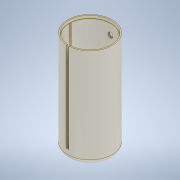
# Autodesk Inventor part: Exterior
Saved by Autodesk Inventor 2020 (Build 240168000, 168)
## iProperties
Created: 2020-10-28
Part Number: Exterior
Material: ABS Plastic
Document SubType Name: Modeling
Designer: aaron
Density: 1.06 g/cm^3
Appearance: Titanium - Polished
Author: aaron
Autodesk Inventor part; units mm, degrees
ref_plane "YZ Plane" through (0, 0, 0) normal (1, 0, 0) x (0, 1, 0)
ref_plane "XZ Plane" through (0, 0, 0) normal (0, 1, 0) x (-1, 0, 0)
ref_plane "XY Plane" through (0, 0, 0) normal (0, 0, 1) x (1, 0, 0)
sketch "Sketch1" plane through (0, 0, 0) normal (0, 0, 1) x (1, 0, 0)
  line L0 (0, 0) -> (35, 0)
  line L1 (45, 10) -> (45, 200)
  line L2 (0, 200) -> (0, 0)
  arc A0 (35, 0) -> (45, 10) centre (35, 10) ccw
  line L3 (41.5, 200) -> (41.5, 10)
  arc A1 (35, 3.5) -> (41.5, 10) centre (35, 10) ccw
  line L4 (35, 3.5) -> (0, 3.5)
  line L5 (41.5, 200) -> (45, 200)
  line L6 (0, 3.5) -> (0, 0)
  point P0 (45, 0)
  dimension "d0" = 90
  dimension "d1" = 200
  dimension "d2" = 10
  dimension "d5" = 3.5
  dimension "d6" = 3.5
  constraints: 14 end point, 4 point on circle, 3 point on line, 2 centre point, 2 horizontal, 2 perpendicular, 2 tangent, 2 vertical, 1 other
  measures "d0" diameter of L1 L2
  measures "d1" distance of point (45, 0) L1.end
  measures "d2" radius of A0
  measures "d5" distance between parallel lines of L0 L4
  measures "d6" distance between parallel lines of L1 L3
revolve "Revolution1" add sketch "Sketch1" angle 360 about axis through (0, 200, 0) along (0, -1, 0)
sketch "Sketch2" plane through (0, 200, 0) normal (0, 1, 0) x (1, 0, 0)
  circle A0 centre (0, 0) radius 45 construction
  line L0 (0, 45) -> (0, -45) construction
  line L1 (-45, 0) -> (45, 0) construction
  circle A1 centre (0, 0) radius 45 construction
  circle A2 centre (0, 0) radius 41.5 construction
  circle A3 centre (0, 0) radius 41.5 construction
  circle A4 centre (0, 0) radius 45 construction
  line L2 (0, -41.5) -> (0, -45) construction
  line L3 (-2.5, -45.45) -> (2.5, -45.45)
  line L4 (2.5, -45.45) -> (2.5, -41.05)
  line L5 (2.5, -41.05) -> (-2.5, -41.05)
  line L6 (-2.5, -41.05) -> (-2.5, -45.45)
  line L7 (-2.5, -45.45) -> (2.5, -41.05) construction
  line L8 (2.5, -45.45) -> (-2.5, -41.05) construction
  point P0 (0, -43.25)
  dimension "d8" = 5
  dimension "d9" = 4.4
  constraints: 18 end point, 4 point on circle, 3 midpoint, 2 parallel, 2 perpendicular, 1 collinear, 1 point on line, 1 vertical, 1 vertical alignment, 1 other
  measures "d8" distance of L3.start L3.end
  measures "d9" distance of L3.end L4.end
extrude "Extrusion1" cut sketch "Sketch2" against normal blind 180
fillet "Fillet1" radius 1 2 edges at (-2.5, 200, 43.1776) (2.5, 200, 43.1776)
sketch "Sketch3" plane through (0, 200, 0) normal (0, 1, 0) x (1, 0, 0)
  arc A0 (3.5, -41.3521) -> (-3.5, -41.3521) centre (0, 0) ccw projected
  circle A1 centre (0, 0) radius 42.5
  circle A2 centre (0, 0) radius 41.5
  point P0 (3.5, -41.3521)
  point P1 (-3.5, -41.3521)
  dimension "d13" = 85
  constraints: 2 centre point, 2 coincident, 1 concentric
  measures "d13" diameter of A1
extrude "Extrusion2" cut sketch "Sketch3" against normal blind 5
ref_plane "Work Plane1" through (0, 200, -45) normal (0, 0, -1) x (-1, 0, 0)
sketch "Sketch4" plane through (0, 200, -45) normal (0, 0, -1) x (-1, 0, 0)
  line L0 (-45, 0) -> (45, 0) construction
  line L1 (0, 0) -> (0, -25) construction
  circle A0 centre (0, -25) radius 5
  point P0 (0, -200)
  point P1 (3.5, 0)
  point P2 (-3.5, 0)
  dimension "d16" = 25
  dimension "d17" = 10
  constraints: 2 end point, 1 centre point, 1 coincident, 1 midpoint, 1 vertical
  measures "d16" distance of L1.start L1.end
  measures "d17" diameter of A0
extrude "Extrusion3" cut sketch "Sketch4" against normal up to surface round surface about axis through (0, 105, 0) along (0, -1, 0) radius 41.5 far side no
sketch "Sketch5" plane through (0, 195, 0) normal (0, 1, 0) x (1, 0, 0)
  line L0 (2.5, -42.4264) -> (2.5, -41.4246) construction
  arc A0 (2.5, -42.4264) -> (-2.5, -42.4264) centre (0, 0) ccw construction
  line L1 (-2.5, -41.4246) -> (-2.5, -42.4264) construction
  arc A1 (2.5, -41.4246) -> (-2.5, -41.4246) centre (0, 0) ccw projected
  arc A2 (2.5, -41.4246) -> (-2.5, -41.4246) centre (0, 0) ccw construction
  line L2 (41.5, 0) -> (-41.5, 0) construction
  line L3 (41.5, 0) -> (39.5, 0)
  arc A3 (39.5, 0) -> (39.4459, 2.0673) centre (0, 0) ccw
  line L4 (41.5, 0) -> (39.5, 0)
  line L5 (0, 0) -> (41.5, 0) construction
  line L6 (0, 0) -> (41.4431, 2.1719) construction
  line L7 (41.4431, 2.1719) -> (39.4459, 2.0673)
  line L8 (0, 41.5) -> (0, -41.5) construction
  arc A4 (41.5, 0) -> (41.4431, 2.1719) centre (0, 0) ccw
  arc A5 (-2.5, -41.4246) -> (2.5, -41.4246) centre (0, 0) ccw
  line L9 (-41.5, 0) -> (-39.5, 0)
  arc A6 (-39.4459, 2.0673) -> (-39.5, 0) centre (0, 0) ccw
  line L10 (-41.4431, 2.1719) -> (-39.4459, 2.0673)
  arc A7 (-41.4431, 2.1719) -> (-41.5, 0) centre (0, 0) ccw
  point P0 (-41.5, 0)
  dimension "d20" = 2
  dimension "d21" = 3
  constraints: 19 end point, 14 point on circle, 5 centre point, 4 point on line, 3 coincident, 3 symmetric about line, 1 horizontal, 1 vertical, 2 other
  measures "d20" distance of L3.end L2.start
  measures "d21" angle of L2 L6
extrude "Extrusion4" add sketch "Sketch5" against normal blind 170 contours L3 A3 L7 A1 | A1 L10 A6 L9
body "Solid1"
